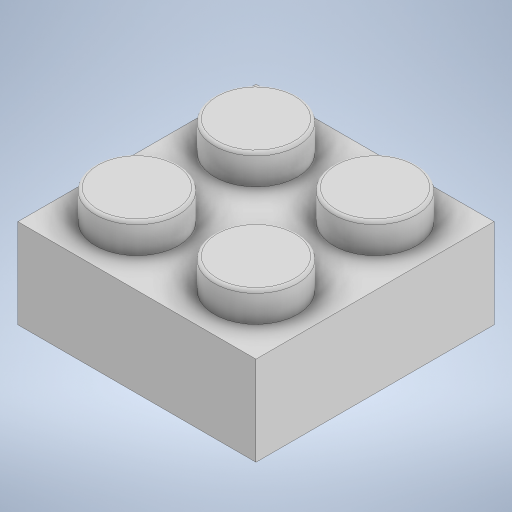
# Autodesk Inventor part: Tercer examen. Cubo LEGO. Villegas
Saved by Autodesk Inventor 2023 (Build 270158000, 158)
## iProperties
Created: 2022-11-04
Part Number: Tercer examen. Cubo LEGO. Villegas
Material: Generic
Document SubType Name: Modeling
Designer: al180794
Density: 1 g/cm^3
Appearance: Default
Author: al180794
Autodesk Inventor part; units mm, degrees
ref_plane "YZ Plane" through (0, 0, 0) normal (1, 0, 0) x (0, 1, 0)
ref_plane "XZ Plane" through (0, 0, 0) normal (0, 1, 0) x (-1, 0, 0)
ref_plane "XY Plane" through (0, 0, 0) normal (0, 0, 1) x (1, 0, 0)
sketch "Sketch2" plane through (0, 0, 0) normal (0, 1, 0) x (-1, 0, 0)
  line L0 (-20, 20) -> (20, 20)
  line L1 (20, 20) -> (20, -20)
  line L2 (20, -20) -> (-20, -20)
  line L3 (-20, -20) -> (-20, 20)
  circle A0 centre (10, 10) radius 7
  circle A1 centre (10, -10) radius 7
  circle A2 centre (-10, -10) radius 7
  circle A3 centre (-10, 10) radius 7
  point P0 (0, 0)
  constraints: 8 end point, 4 centre point, 2 parallel, 1 horizontal, 1 perpendicular
extrude "Extrusion1" add sketch "Sketch2" along normal blind 5 and the other way blind 10
extrude "Extrusion2" add sketch "Sketch2" along normal blind 10 and the other way blind 5 contours A0 | A1 | A2 | A3
fillet "Fillet1" radius 0.5 4 edges at (-3, 10, 10) (-3, 10, -10) (17, 10, -10) (17, 10, 10)
body "Solid1"
